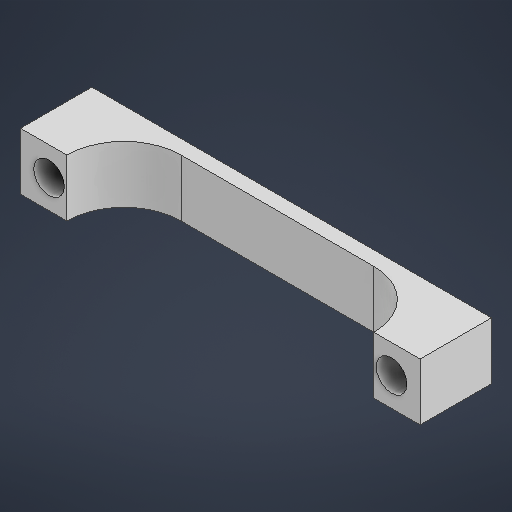
# Autodesk Inventor part: Ultrasonic_sensor_frame_Top
Saved by Autodesk Inventor 2026.1 (Build 301233020, 233B)
## iProperties
Created: 2025-10-28
Part Number: Ultrasonic_sensor_frame_Top
Material: Generic
Document SubType Name: Modeling
Designer: Asus
Density: 1 g/cm^3
Appearance: Default
Author: Asus
Autodesk Inventor part; units mm, degrees
ref_plane "YZ Plane" through (0, 0, 0) normal (1, 0, 0) x (0, 1, 0)
ref_plane "XZ Plane" through (0, 0, 0) normal (0, 1, 0) x (-1, 0, 0)
ref_plane "XY Plane" through (0, 0, 0) normal (0, 0, 1) x (1, 0, 0)
sketch "Sketch1" plane through (0, 0, 0) normal (0, 1, 0) x (-1, 0, 0)
  line L0 (0, 0) -> (-27, 0) construction
  line L1 (-27, -8) -> (0, -8)
  arc A0 (0, -8) -> (0, 8) centre (0, 0) ccw
  arc A1 (-27, 8) -> (-27, -8) centre (-27, 0) ccw
  line L2 (14.5, 10) -> (-41.5, 10)
  line L3 (-41.5, 10) -> (-41.5, -10)
  line L4 (-41.5, -10) -> (14.5, -10)
  line L5 (14.5, -10) -> (14.5, 10)
  line L6 (14.5, 10) -> (-41.5, -10) construction
  line L7 (-41.5, 10) -> (14.5, -10) construction
  line L8 (14.5, 10) -> (-41.5, 10)
  line L9 (-41.5, 10) -> (-41.5, 15)
  line L10 (-41.5, 15) -> (14.5, 15)
  line L11 (14.5, 15) -> (14.5, 10)
  arc A2 (0, -8) -> (-5.3358, 5.9607) centre (0, 0) ccw
  arc A3 (-21.6642, 5.9607) -> (-27, -8) centre (-27, 0) ccw
  line L12 (9, -10) -> (-36, -10)
  line L13 (-36, -10) -> (-36, 10) construction
  line L14 (-36, 10) -> (9, 10)
  line L15 (9, 10) -> (9, -10) construction
  line L16 (9, -10) -> (-36, 10) construction
  line L17 (-36, -10) -> (9, 10) construction
  line L18 (9, 10) -> (-6, 10)
  line L19 (-6, 10) -> (-6, 5.9607)
  line L20 (-36, 10) -> (-21, 10)
  line L21 (-21, 10) -> (-21, 5.9607)
  line L22 (-5.3358, 5.9607) -> (-21.6642, 5.9607) construction
  line L23 (-21, 5.9607) -> (-21.6642, 5.9607)
  line L24 (-6, 5.9607) -> (-5.3358, 5.9607)
  point P0 (-13.5, 0)
  point P1 (-27, 8)
  point P2 (0, 8)
  dimension "d0" = 27
  dimension "d1" = 16
  dimension "d2" = 56
  dimension "d3" = 20
  dimension "d4" = 5
  dimension "d5" = 45
  dimension "d6" = 15
  dimension "d7" = 15
  constraints: 52 end point, 8 point on circle, 6 parallel, 6 perpendicular, 5 midpoint, 5 point on line, 4 centre point, 4 horizontal, 2 coincident, 2 collinear, 2 tangent, 1 concentric
  measures "d0" distance of L0.start L0.end
  measures "d1" diameter of A1
  measures "d2" distance of L4.end L3.end
  measures "d3" distance of L3.end L2.end
  measures "d4" distance of L8.end L9.end
  measures "d5" distance of L13.end L14.end
  measures "d6" distance of L14.end L18.end
  measures "d7" distance of L13.end L20.end
extrude "Extrusion1" add sketch "Sketch1" along normal blind 8 contours L1 A0 A2 L24 L19 L2 L5 L4 L3 L21 L23 A3 A1
extrude "Extrusion2" add sketch "Sketch1" along normal blind 15.5 contours L2 L9 L10 L11
sketch "Sketch2" plane through (21, 0, 10) normal (0, 0, -1) x (-1, 0, 0)
  line L0 (35.5, 8) -> (15, 8) projected
  line L1 (-20.5, 8) -> (-20.5, 15.5) projected
  line L2 (35.5, 8) -> (-20.5, 8)
  line L3 (-20.5, 8) -> (-20.5, 15.5)
  line L4 (-20.5, 15.5) -> (35.5, 15.5)
  line L5 (35.5, 15.5) -> (35.5, 8)
  line L6 (31, 8) -> (-16, 8)
  line L7 (-16, 8) -> (-16, 12.5)
  line L8 (-16, 12.5) -> (31, 12.5)
  line L9 (31, 12.5) -> (31, 8)
  line L10 (-20.5, 8) -> (35.5, 8) projected
  point P0 (21, 0)
  point P1 (7.5, 8)
  dimension "d12" = 47
  dimension "d13" = 4.5
  constraints: 16 end point, 4 parallel, 2 horizontal, 2 midpoint, 2 perpendicular, 1 point on line
  measures "d12" distance of L7.end L8.end
  measures "d13" distance of L6.end L7.end
extrude "Extrusion3" add sketch "Sketch2" along normal blind 3 contours L0 L9 L8 L7 L2 L1 L4 L5
sketch "Sketch3" plane through (41.5, 0, -10) normal (0, 0, -1) x (-1, 0, 0)
  circle A0 centre (52, 4) radius 2.15
  line L0 (56, 0) -> (56, 8) projected
  line L1 (0, 0) -> (56, 0) projected
  circle A1 centre (4, 4) radius 2.15
  line L2 (0, 0) -> (0, 8) projected
  point P0 (41.5, 0)
  dimension "d16" = 4.3
  dimension "d17" = 4
  dimension "d18" = 4
  dimension "d19" = 4.3
  dimension "d20" = 4
  dimension "d21" = 4
  constraints: 2 centre point
  measures "d16" diameter of A0
  measures "d17" distance from line of L0 A0.centre
  measures "d18" distance from line of L1 A0.centre
  measures "d19" diameter of A1
  measures "d20" distance from line of L2 A1.centre
  measures "d21" distance from line of L1 A1.centre
extrude "Extrusion4" cut sketch "Sketch3" against normal blind 32
sketch "Sketch4" plane through (-14.5, 0, 15) normal (0, 0, 1) x (1, 0, 0)
  circle A0 centre (4, 12) radius 1.95
  circle A1 centre (4, 4) radius 2.15 projected
  line L0 (0, 0) -> (0, 15.5) projected
  circle A2 centre (52, 12) radius 1.95
  circle A3 centre (52, 4) radius 2.15 projected
  line L1 (56, 0) -> (56, 15.5) projected
  line L2 (0, 15.5) -> (56, 15.5) projected
  point P0 (14.5, 0)
  dimension "d24" = 3.9
  dimension "d25" = 8
  dimension "d26" = 4
  dimension "d27" = 3.9
  dimension "d28" = 8
  dimension "d29" = 4
  dimension "d30" = 3.5
  dimension "d31" = 3.5
  constraints: 2 centre point
  measures "d24" diameter of A0
  measures "d25" distance of A1.centre A0.centre
  measures "d26" distance from line of L0 A0.centre
  measures "d27" diameter of A2
  measures "d28" distance of A3.centre A2.centre
  measures "d29" distance from line of L1 A2.centre
  measures "d30" distance from line of L2 A2.centre
  measures "d31" distance from line of L2 A0.centre
extrude "Extrusion5" add sketch "Sketch4" along normal blind 2 contours A0 | A2
sketch "Sketch5" plane through (0, 15.5, 0) normal (0, 1, 0) x (1, 0, 0)
  line L0 (-14.5, 10) -> (-14.5, -7) projected
  line L1 (-14.5, 0) -> (41.5, 0)
  line L2 (41.5, 0) -> (41.5, -17)
  line L3 (41.5, -17) -> (-14.5, -17)
  line L4 (-14.5, -17) -> (-14.5, 0)
  point P0 (0, 0)
  dimension "d34" = 17
  constraints: 8 end point, 2 parallel, 1 horizontal, 1 perpendicular, 1 point on line
  measures "d34" distance of L1.end L2.end
extrude "Extrusion6" cut sketch "Sketch5" against normal blind 27
body "Solid1"
